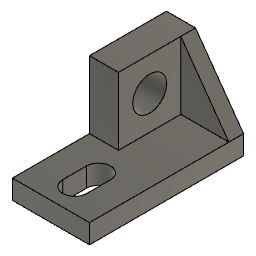
Figure-2 (Autodesk Fusion 360 design; units mm, degrees)
Autodesk Fusion 360 part; units mm, degrees
sketch "Sketch2" plane through (0, 0, 0) normal (0, 0, 1) x (1, 0, 0)
  line L0 (25.4, 50.8) -> (-25.4, 50.8)
  line L1 (-25.4, 50.8) -> (-25.4, -50.8)
  line L2 (-25.4, -50.8) -> (25.4, -50.8)
  line L3 (25.4, -50.8) -> (25.4, 50.8)
  line L4 (25.4, 50.8) -> (-25.4, -50.8) construction
  line L5 (-25.4, 50.8) -> (25.4, -50.8) construction
  dimension "d3" = 50.8
  dimension "d4" = 101.6
  constraint horizontal L0
  constraint perpendicular L0 L1
  constraint parallel L0 L2
  constraint parallel L1 L3
  constraint coincident L4 origin
  constraint coincident L5 origin
  measures "d3" distance of L1.end L2.end
  measures "d4" distance of L0.end L1.end
extrude "Extrude1" add sketch "Sketch2" along normal blind 57.2
sketch "Sketch3" plane through (0, 0, 57.2) normal (0, 0, 1) x (-1, 0, 0)
  line L0 (-25.4, 50.8) -> (-25.4, -50.8)
  line L1 (-25.4, -50.8) -> (25.4, -50.8)
  line L2 (25.4, -50.8) -> (25.4, 50.8)
  line L3 (25.4, 50.8) -> (-25.4, 50.8)
  line L4 (25.4, -50.8) -> (-25.4, -50.8)
  line L5 (-25.4, -50.8) -> (-25.4, 50.8)
  line L6 (-25.4, 50.8) -> (25.4, 50.8)
  line L7 (25.4, 50.8) -> (25.4, -50.8)
  line L8 (25.4, -50.8) -> (-25.4, 50.8) construction
  line L9 (-25.4, -50.8) -> (25.4, 50.8) construction
  constraint horizontal L4
  constraint perpendicular L4 L5
  constraint parallel L4 L6
  constraint parallel L5 L7
  constraint coincident L1.end L2.start
  constraint coincident L8 origin
  constraint coincident L9 origin
extrude "Extrude2" cut sketch "Sketch3" against normal blind 44.5
sketch "Sketch4" plane through (0, 0, 0) normal (0, 0, 1) x (1, 0, 0)
  line L0 (-25.4, 50.8, 12.7) -> (-6.3, 50.8, 12.7)
  line L1 (-6.3, 50.8, 12.7) -> (-6.3, 0, 12.7)
  line L2 (-6.3, 0, 12.7) -> (-25.4, 0, 12.7)
  line L3 (-25.4, 0, 12.7) -> (-25.4, 50.8, 12.7)
  point P0 (-25.4, 50.8)
  dimension "d9" = 19.1
  dimension "d10" = 50.8
extrude "Extrude3" add sketch "Sketch4" along normal blind 44.5 contours L0 L1 L2 L3 in plane through (0, 0, 12.7) normal (0, 0, 1)
sketch "Sketch5" plane through (0, 0, 12.7) normal (0, 0, 1) x (-1, 0, 0)
  line L0 (6.3, -50.8) -> (6.3, 0)
  line L1 (6.3, 0) -> (25.4, 0)
  line L2 (25.4, 0) -> (25.4, 50.8)
  line L3 (25.4, 50.8) -> (-25.4, 50.8)
  line L4 (-25.4, 50.8) -> (-25.4, -50.8)
  line L5 (-25.4, -50.8) -> (6.3, -50.8)
  line L6 (-25.4, -50.8, 0) -> (6.3, -50.8, 44.5)
  line L7 (6.3, -50.8, 44.5) -> (6.3, -50.8, 0)
  point P0 (6.3, -50.8)
  constraint coincident L4.end L5.start
  constraint coincident P0 L0.start
extrude "Extrude4" add sketch "Sketch5" along normal blind 9.7 contours L5 L6 L7 in plane through (0, 50.8, 12.7) normal (0, -1, 0)
sketch "Sketch11" plane through (0, 0, 12.7) normal (0, 0, 1) x (-1, 0, 0)
  line L0 (-7.9, 35.1) -> (-7.9, 19.4)
  arc A0 (-7.9, 19.4) -> (7.9, 19.4) centre (0, 19.4) ccw
  line L1 (7.9, 19.4) -> (7.9, 35.1)
  arc A1 (7.9, 35.1) -> (-7.9, 35.1) centre (0, 35.1) ccw
  point P0 (0, 50.8)
  point P1 (0, 35.1)
  point P2 (0, 19.4)
  constraint vertical P0 A1.centre
  constraint vertical P1 A0.centre
  constraint parallel L0 L1
  constraint coincident P2 A0.centre
  constraint coincident P1 A1.centre
extrude "Extrude5" cut sketch "Sketch11" against normal blind 40
sketch "Sketch12" plane through (-6.3, 0, 0) normal (1, 0, 0) x (0, 1, 0)
  line L0 (41.1, 12.7) -> (41.1, 57.2)
  line L1 (41.1, 57.2) -> (0, 57.2)
  line L2 (0, 57.2) -> (0, 12.7)
  line L3 (0, 12.7) -> (41.1, 12.7)
  circle A0 centre (20.6, 34.8) radius 11.175
extrude "Extrude6" cut sketch "Sketch12" against normal blind 90 contours A0
